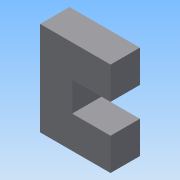
# Autodesk Inventor part: stopper
Saved by Autodesk Inventor 2015 (Build 190159000, 159)
## iProperties
Created: 2014-09-02
Part Number: stopper
Material: Generic
Document SubType Name: Modeling
Designer: shohei
Density: 1 g/cm^3
Appearance: Default
Author: shohei
Autodesk Inventor part; units mm, degrees
ref_plane "YZ Plane" through (0, 0, 0) normal (1, 0, 0) x (0, 1, 0)
ref_plane "XZ Plane" through (0, 0, 0) normal (0, 1, 0) x (-1, 0, 0)
ref_plane "XY Plane" through (0, 0, 0) normal (0, 0, 1) x (1, 0, 0)
sketch "Sketch1" plane through (0, 0, 0) normal (0, 1, 0) x (-1, 0, 0)
  line L0 (0, 0) -> (12, 0)
  line L1 (12, 0) -> (12, 16)
  line L2 (12, 16) -> (0, 16)
  line L3 (0, 16) -> (0, 0)
  line L4 (0, 5.5) -> (6.5385, 5.5)
  line L5 (6.5385, 5.5) -> (6.5385, 10.5)
  line L6 (6.5385, 10.5) -> (0, 10.5)
  line L7 (0, 10.5) -> (0, 5.5)
  line L8 (7.6283, 8) -> (-1.5257, 8)
  dimension "d2" = 5
  dimension "d3" = 12
  dimension "d4" = 8
  dimension "d5" = 16
  constraints: 18 end point, 4 parallel, 3 horizontal, 2 perpendicular, 1 point on line, 1 other
  measures "d2" distance of L4.end L5.end
  measures "d3" distance of L1.end L2.end
  measures "d4" distance between parallel lines of L2 L8
  measures "d5" distance of L0.end L1.end
extrude "Extrusion1" add sketch "Sketch1" along normal blind 5 contours L3 L4 L5 L6 L2 L1 L0
body "Solid1"
